Autodesk Fusion 360 part; units mm, degrees
(part 3 of 3)
  spline S21 degree 5 poles (6.5893, -10.3268) (6.5899, -10.3186) (6.5909, -10.3022) (6.5925, -10.2777) (6.5944, -10.245) (6.5965, -10.2042) (6.5984, -10.1634) (6.6, -10.1228) (6.6014, -10.0821) (6.6026, -10.0416) (6.6036, -10.0012) (6.6042, -9.9608) (6.6047, -9.9205) (6.6049, -9.8802) (6.6049, -9.8401) (6.6046, -9.8) (6.604, -9.76) (6.6033, -9.7202) (6.6022, -9.6803) (6.601, -9.6406) (6.5994, -9.601) (6.5977, -9.5615) (6.5957, -9.522) (6.5934, -9.4827) (6.5909, -9.4434) (6.5881, -9.4043) (6.585, -9.3652) (6.5818, -9.3263) (6.5782, -9.2875) (6.5744, -9.2487) (6.5703, -9.2101) (6.566, -9.1716) (6.5614, -9.1332) (6.5566, -9.095) (6.5515, -9.0568) (6.5461, -9.0188) (6.5404, -8.9809) (6.5345, -8.9431) (6.5283, -8.9054) (6.5218, -8.8679) (6.5151, -8.8305) (6.5081, -8.7933) (6.5007, -8.7562) (6.4931, -8.7193) (6.4852, -8.6825) (6.4771, -8.6458) (6.4686, -8.6093) (6.4599, -8.573) (6.4508, -8.5368) (6.4415, -8.5008) (6.4318, -8.4649) (6.4218, -8.4293) (6.4115, -8.3938) (6.4009, -8.3585) (6.3899, -8.3235) (6.3786, -8.2886) (6.367, -8.2539) (6.355, -8.2194) (6.3428, -8.185) (6.3303, -8.1509) (6.3173, -8.1171) (6.3038, -8.0836) (6.2898, -8.0504) (6.2753, -8.0175) (6.2604, -7.9849) (6.2451, -7.9526) (6.2295, -7.9205) (6.2138, -7.8885) (6.1976, -7.8568) (6.1809, -7.8255) (6.1631, -7.795) (6.1477, -7.7714) (6.1354, -7.7542) (6.1269, -7.743) (6.1225, -7.7374) knots -1 -1 -1 -1 -1 -1 -0.98571429 -0.97142857 -0.95714286 -0.94285714 -0.92857143 -0.91428571 -0.9 -0.88571429 -0.87142857 -0.85714286 -0.84285714 -0.82857143 -0.81428571 -0.8 -0.78571429 -0.77142857 -0.75714286 -0.74285714 -0.72857143 -0.71428571 -0.7 -0.68571429 -0.67142857 -0.65714286 -0.64285714 -0.62857143 -0.61428571 -0.6 -0.58571429 -0.57142857 -0.55714286 -0.54285714 -0.52857143 -0.51428571 -0.5 -0.48571429 -0.47142857 -0.45714286 -0.44285714 -0.42857143 -0.41428571 -0.4 -0.38571429 -0.37142857 -0.35714286 -0.34285714 -0.32857143 -0.31428571 -0.3 -0.28571429 -0.27142857 -0.25714286 -0.24285714 -0.22857143 -0.21428571 -0.2 -0.18571429 -0.17142857 -0.15714286 -0.14285714 -0.12857143 -0.11428571 -0.1 -0.08571429 -0.07142857 -0.05714286 -0.04285714 -0.02857143 -0.01428571 0 0 0 0 0 0
  line L21 (6.1225, -7.7374) -> (5.7679, -7.2884)
  arc A43 (5.8518, -5.9553) -> (5.7679, -7.2884) centre (6.5526, -6.6686) ccw
  arc A44 (5.8518, -5.9553) -> (5.9553, -5.8518) centre (0, 0) ccw
  arc A45 (7.2884, -5.7679) -> (5.9553, -5.8518) centre (6.6686, -6.5526) ccw
  line L22 (7.2884, -5.7679) -> (7.7374, -6.1225)
  spline S22 degree 5 poles (7.7374, -6.1225) (7.743, -6.1269) (7.7542, -6.1354) (7.7714, -6.1477) (7.795, -6.1631) (7.8255, -6.1809) (7.8568, -6.1976) (7.8885, -6.2138) (7.9205, -6.2295) (7.9526, -6.2451) (7.9849, -6.2604) (8.0175, -6.2753) (8.0504, -6.2898) (8.0836, -6.3038) (8.1171, -6.3173) (8.1509, -6.3303) (8.185, -6.3428) (8.2194, -6.355) (8.2539, -6.367) (8.2886, -6.3786) (8.3235, -6.3899) (8.3585, -6.4009) (8.3938, -6.4115) (8.4293, -6.4218) (8.4649, -6.4318) (8.5008, -6.4415) (8.5368, -6.4508) (8.573, -6.4599) (8.6093, -6.4686) (8.6458, -6.4771) (8.6825, -6.4852) (8.7193, -6.4931) (8.7562, -6.5007) (8.7933, -6.5081) (8.8305, -6.5151) (8.8679, -6.5218) (8.9054, -6.5283) (8.9431, -6.5345) (8.9809, -6.5404) (9.0188, -6.5461) (9.0568, -6.5515) (9.095, -6.5566) (9.1332, -6.5614) (9.1716, -6.566) (9.2101, -6.5703) (9.2487, -6.5744) (9.2875, -6.5782) (9.3263, -6.5818) (9.3652, -6.585) (9.4043, -6.5881) (9.4434, -6.5909) (9.4827, -6.5934) (9.522, -6.5957) (9.5615, -6.5977) (9.601, -6.5994) (9.6406, -6.601) (9.6803, -6.6022) (9.7202, -6.6033) (9.76, -6.604) (9.8, -6.6046) (9.8401, -6.6049) (9.8802, -6.6049) (9.9205, -6.6047) (9.9608, -6.6042) (10.0012, -6.6036) (10.0416, -6.6026) (10.0821, -6.6014) (10.1228, -6.6) (10.1634, -6.5984) (10.2042, -6.5965) (10.245, -6.5944) (10.2777, -6.5925) (10.3022, -6.5909) (10.3186, -6.5899) (10.3268, -6.5893) knots 0 0 0 0 0 0 0.01428571 0.02857143 0.04285714 0.05714286 0.07142857 0.08571429 0.1 0.11428571 0.12857143 0.14285714 0.15714286 0.17142857 0.18571429 0.2 0.21428571 0.22857143 0.24285714 0.25714286 0.27142857 0.28571429 0.3 0.31428571 0.32857143 0.34285714 0.35714286 0.37142857 0.38571429 0.4 0.41428571 0.42857143 0.44285714 0.45714286 0.47142857 0.48571429 0.5 0.51428571 0.52857143 0.54285714 0.55714286 0.57142857 0.58571429 0.6 0.61428571 0.62857143 0.64285714 0.65714286 0.67142857 0.68571429 0.7 0.71428571 0.72857143 0.74285714 0.75714286 0.77142857 0.78571429 0.8 0.81428571 0.82857143 0.84285714 0.85714286 0.87142857 0.88571429 0.9 0.91428571 0.92857143 0.94285714 0.95714286 0.97142857 0.98571429 1 1 1 1 1 1
  arc A46 (10.3268, -6.5893) -> (10.8699, -5.6486) centre (0, 0) ccw
  spline S23 degree 5 poles (10.8699, -5.6486) (10.8663, -5.6413) (10.859, -5.6265) (10.8481, -5.6045) (10.8334, -5.5752) (10.8148, -5.5388) (10.7961, -5.5026) (10.7772, -5.4665) (10.7581, -5.4307) (10.7388, -5.395) (10.7194, -5.3595) (10.6998, -5.3242) (10.6801, -5.289) (10.6601, -5.2541) (10.64, -5.2193) (10.6197, -5.1848) (10.5993, -5.1504) (10.5787, -5.1163) (10.5579, -5.0823) (10.5369, -5.0485) (10.5158, -5.015) (10.4945, -4.9816) (10.473, -4.9485) (10.4514, -4.9155) (10.4296, -4.8828) (10.4076, -4.8503) (10.3854, -4.818) (10.3631, -4.7859) (10.3406, -4.7541) (10.318, -4.7224) (10.2951, -4.691) (10.2721, -4.6598) (10.249, -4.6289) (10.2256, -4.5982) (10.2021, -4.5677) (10.1785, -4.5375) (10.1546, -4.5075) (10.1306, -4.4777) (10.1064, -4.4482) (10.082, -4.4189) (10.0575, -4.3899) (10.0328, -4.3612) (10.0079, -4.3327) (9.9829, -4.3045) (9.9576, -4.2766) (9.9322, -4.249) (9.9066, -4.2216) (9.8809, -4.1945) (9.855, -4.1677) (9.8289, -4.1411) (9.8026, -4.1149) (9.7761, -4.089) (9.7494, -4.0635) (9.7226, -4.0383) (9.6955, -4.0134) (9.6683, -3.9888) (9.6409, -3.9646) (9.6133, -3.9407) (9.5856, -3.917) (9.5576, -3.8938) (9.5295, -3.871) (9.501, -3.8487) (9.4723, -3.8269) (9.4433, -3.8057) (9.4141, -3.785) (9.3847, -3.7646) (9.3552, -3.7446) (9.3255, -3.7248) (9.2957, -3.7054) (9.2656, -3.6867) (9.2349, -3.6691) (9.2098, -3.6563) (9.1905, -3.6476) (9.1775, -3.6422) (9.171, -3.6396) knots -1 -1 -1 -1 -1 -1 -0.98571429 -0.97142857 -0.95714286 -0.94285714 -0.92857143 -0.91428571 -0.9 -0.88571429 -0.87142857 -0.85714286 -0.84285714 -0.82857143 -0.81428571 -0.8 -0.78571429 -0.77142857 -0.75714286 -0.74285714 -0.72857143 -0.71428571 -0.7 -0.68571429 -0.67142857 -0.65714286 -0.64285714 -0.62857143 -0.61428571 -0.6 -0.58571429 -0.57142857 -0.55714286 -0.54285714 -0.52857143 -0.51428571 -0.5 -0.48571429 -0.47142857 -0.45714286 -0.44285714 -0.42857143 -0.41428571 -0.4 -0.38571429 -0.37142857 -0.35714286 -0.34285714 -0.32857143 -0.31428571 -0.3 -0.28571429 -0.27142857 -0.25714286 -0.24285714 -0.22857143 -0.21428571 -0.2 -0.18571429 -0.17142857 -0.15714286 -0.14285714 -0.12857143 -0.11428571 -0.1 -0.08571429 -0.07142857 -0.05714286 -0.04285714 -0.02857143 -0.01428571 0 0 0 0 0 0
  line L23 (9.171, -3.6396) -> (8.6393, -3.428)
  arc A47 (8.0454, -2.2316) -> (8.6393, -3.428) centre (9.0091, -2.4989) ccw
  circle A48 centre (0, 0) radius 4.4
  dimension "d21" = 8.8
  constraint coincident A0.centre A2.centre
  measures "d21" diameter of A48
extrude "Extrude6" add sketch "Sketch6" along normal blind 0.5 contours A48 in component "Spur Gear (12 teeth)"
sketch "Sketch7" plane through (0, 0, -2) normal (0, 0, -1) x (-1, 0, 0)
  arc A0 (3.5, 4.8734) -> (-3.5, 4.8734) centre (0, 0) ccw
  line L0 (-3.5, 4.8734) -> (-3.5, -2.6)
  line L1 (-3.5, -2.6) -> (-1.5, -4.6)
  line L2 (-1.5, -4.6) -> (1.5, -4.6)
  line L3 (1.5, -4.6) -> (3.5, -2.6)
  line L4 (3.5, -2.6) -> (3.5, 4.8734)
  line L5 (-2.75, -1.5877) -> (0, -3.1754)
  line L6 (0, -3.1754) -> (2.75, -1.5877)
  line L7 (2.75, -1.5877) -> (2.75, 1.5877)
  line L8 (2.75, 1.5877) -> (0, 3.1754)
  line L9 (0, 3.1754) -> (-2.75, 1.5877)
  line L10 (-2.75, 1.5877) -> (-2.75, -1.5877)
  circle A1 centre (0, 0) radius 2.75 construction
  dimension "d24" = 5.5
  constraint coincident A0.centre A1.centre
  constraint tangent L10 A1
  constraint vertical L7
  measures "d24" diameter of A1
extrude "Extrude7" cut sketch "Sketch7" against normal blind 4 contours L5 L6 L7 L8 L9 L10 in component "Spur Gear (12 teeth)"
sketch "Sketch8" plane through (0, 0, 2) normal (0, 0, -1) x (-1, 0, 0)
  line L0 (-2.75, 1.5877) -> (-2.75, -1.5877)
  line L1 (-2.75, -1.5877) -> (0, -3.1754)
  line L2 (0, -3.1754) -> (2.75, -1.5877)
  line L3 (2.75, -1.5877) -> (2.75, 1.5877)
  line L4 (2.75, 1.5877) -> (0, 3.1754)
  line L5 (0, 3.1754) -> (-2.75, 1.5877)
  circle A0 centre (0, 0) radius 1.5
  dimension "d27" = 3
  constraint coincident A0.centre origin
  measures "d27" diameter of A0
extrude "Extrude8" cut sketch "Sketch8" against normal blind 18 contours A0 in component "Spur Gear (12 teeth)"
chamfer "Chamfer1" distance 0.5 angle 45 6 edges at (1.375, 2.3816, -2) (-1.375, 2.3816, -2) (-2.75, 0, -2) (-1.375, -2.3816, -2) (1.375, -2.3816, -2) (2.75, 0, -2) in component "Spur Gear (12 teeth)"
sketch "Sketch9" plane through (0, 0, 6.5) normal (0, 0, 1) x (1, 0, 0)
  circle A0 centre (0, 0) radius 1.5
  circle A1 centre (0, 0) radius 4.4
  circle A2 centre (0, 0) radius 4
  line L0 (-3, 2.6458) -> (-3, -2.6458)
  line L1 (3, -2.6458) -> (3, 2.6458)
  line L2 (-3, 0) -> (3, 0) construction
  line L3 (3, -2.6458) -> (0, -4)
  line L4 (-3, -2.6458) -> (0, -4)
  dimension "d31" = 8
  dimension "d32" = 6
  constraint concentric A0 A2
  constraint coincident A2 L0.start
  constraint vertical L0
  constraint coincident A2 L1.end
  constraint coincident L0 L2.start
  constraint coincident L1 L2.end
  constraint perpendicular L1 L2
  constraint midpoint A0.centre L2
  constraint coincident A2 L1.start
  constraint coincident A2 L0.end
  constraint coincident A2 L3.end
  constraint equal L3 L4
  measures "d31" diameter of A2
  measures "d32" distance of L0 L1
extrude "Extrude9" cut sketch "Sketch9" against normal blind 2 contours A2 L0 L1 L3 L4 in component "Spur Gear (12 teeth)"
extrude "Extrude10" add 1 faces at (1.1667, -2.0207, 2) along direction (0, 0, -1) blind 0.7 in component "Spur Gear (12 teeth)"
component "Spur Gear (12 teeth)" placed x (1, 0, 0) y (0, 1, 0) z (0, 0, 1) at (0, 0, 0)
